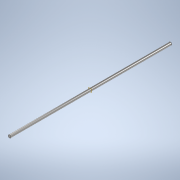
# Autodesk Inventor part: 8mm smooth rod
Saved by Autodesk Inventor 2020.4 (Build 244396000, 396)
## iProperties
Created: 2021-03-01
Part Number: 8mm smooth rod
Material: Stainless Steel, 440C
Document SubType Name: Modeling
Designer: AOB
Mass: 179.196 g
Surface Area: 116.616 cm^2
Volume: 23.1221 cm^3
Density: 7.75 g/cm^3
Appearance: Semi-Polished
Author: AOB
Autodesk Inventor part; units mm, degrees
ref_plane "YZ Plane" through (0, 0, 0) normal (1, 0, 0) x (0, 1, 0)
ref_plane "XZ Plane" through (0, 0, 0) normal (0, 1, 0) x (-1, 0, 0)
ref_plane "XY Plane" through (0, 0, 0) normal (0, 0, 1) x (1, 0, 0)
sketch "Sketch1" plane through (0, 0, 0) normal (0, 0, 1) x (1, 0, 0)
  circle A0 centre (0, 0) radius 4
  dimension "d0" = 8
  constraints: 1 centre point, 1 coincident
  measures "d0" diameter of A0
extrude "Extrusion1" add sketch "Sketch1" along normal blind 460
ref_plane "Work Plane1" through (0, 0, 230) normal (0, 0, 1) x (1, 0, 0)
body "Solid1"
